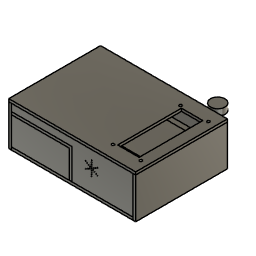
nfc_box (Autodesk Fusion 360 design; units mm, degrees)
Autodesk Fusion 360 part; units mm, degrees
note: some values were not read from the file. Chosen so that the rebuilt part matches the saved one: which bodies a step acts on. Set by a fixed rule: which sketch regions a step uses.
(part 1 of 2)
sketch "Sketch2" plane through (0, 0, 0) normal (0, 0, 1) x (1, 0, 0)
  line L0 (0, 0) -> (80, 0)
  line L1 (80, 0) -> (80, 36)
  line L2 (80, 36) -> (0, 36)
  line L3 (0, 36) -> (0, 0)
  line L4 (0, 0) -> (2.5, 0)
  line L5 (2.5, 0) -> (2.5, 2.5)
  line L6 (0, 0) -> (0, 5.6)
  line L7 (4.6, 5.6) -> (75.4, 5.6)
  line L8 (75.4, 5.6) -> (75.4, 29.4)
  line L9 (75.4, 29.4) -> (4.6, 29.4)
  line L10 (4.6, 29.4) -> (4.6, 5.6)
  circle A0 centre (2.5, 2.5) radius 1.5
  line L11 (0, 36) -> (2.5, 36)
  line L12 (80, 36) -> (77.5, 36)
  line L13 (80, 0) -> (80, 2.5)
  circle A1 centre (77.5, 33.5) radius 1.5
  circle A2 centre (77.5, 2.5) radius 1.5
  circle A3 centre (2.5, 33.5) radius 1.5
  line L14 (5.5434, 32.3445) -> (47.974, 32.3445)
  line L15 (47.974, 32.3445) -> (47.974, 35.1607)
  line L16 (47.974, 35.1607) -> (5.5434, 35.1607)
  line L17 (5.5434, 35.1607) -> (5.5434, 32.3445)
  dimension "d5" = 80
  dimension "d6" = 36
  dimension "d7" = 2.5
  dimension "d8" = 2.5
  dimension "d10" = 5.6
  dimension "d11" = 4.6
  dimension "d12" = 70.8
  dimension "d13" = 23.8
  dimension "d14" = 3
  dimension "d15" = 2.5
  dimension "d16" = 2.5
  dimension "d17" = 2.5
  dimension "d18" = 2.5
  dimension "d19" = 2.5
  dimension "d20" = 2.5
  dimension "d21" = 3
  dimension "d22" = 3
  dimension "d23" = 3
  constraint horizontal L0
  constraint vertical L1
  constraint horizontal L2
  constraint vertical L3
  constraint coincident L0.start L3.end
  constraint perpendicular L3 L4
  constraint perpendicular L4 L5
  constraint perpendicular L4 L6
  constraint horizontal L7
  constraint vertical L8
  constraint horizontal L9
  constraint vertical L10
  constraint coincident L5.end A0.centre
  constraint perpendicular L3 L11
  constraint perpendicular L1 L12
  constraint perpendicular L0 L13
  constraint horizontal L14
  constraint vertical L15
  constraint horizontal L16
  constraint vertical L17
  measures "d5" distance of L0.start L0.end
  measures "d6" distance of L0.start L2.end
  measures "d7" distance of L0.start L4.end
  measures "d8" distance of L4.end L5.end
  measures "d10" distance of L0.start L6.end
  measures "d11" distance of L6.end L7.start
  measures "d12" distance of L7.start L7.end
  measures "d13" distance of L7.start L9.end
  measures "d14" diameter of A0
  measures "d15" distance of L2.end L11.end
  measures "d16" distance of L11.end A3.centre
  measures "d17" distance of L1.end L12.end
  measures "d18" distance of L12.end A1.centre
  measures "d19" distance of L0.end L13.end
  measures "d20" distance of L13.end A2.centre
  measures "d21" diameter of A1
  measures "d22" diameter of A2
  measures "d23" diameter of A3
extrude "Extrude1" add sketch "Sketch2" against normal blind 20 contours L14 L15 L16 L17 makes body 1
extrude "Extrude2" add sketch "Sketch2" along normal blind 2 separate body makes body 2
extrude "Extrude3" add sketch "Sketch2" along normal blind 2 contours L14 L15 L16 L17 bodies 1 2
extrude "Extrude4" add sketch "Sketch2" along normal blind 10 contours L7 L8 L9 L10 bodies 1
sketch "Sketch3" plane through (0, 0, 0) normal (0, 0, 1) x (1, 0, 0)
  line L0 (0, 0) -> (0, -10)
  line L1 (0, -10) -> (119.888, -10)
  line L2 (119.888, -10) -> (119.888, -60.038)
  line L3 (119.888, -60.038) -> (0, -60.038)
  line L4 (0, -60.038) -> (0, -10)
  line L5 (0, -10) -> (5.08, -10)
  line L6 (0, -60.038) -> (5.08, -60.038)
  line L7 (119.888, -10) -> (114.808, -10)
  line L8 (119.888, -60.038) -> (114.808, -60.038)
  circle A0 centre (114.808, -54.958) radius 1.778
  circle A1 centre (114.808, -15.08) radius 1.75
  circle A2 centre (5.08, -15.08) radius 1.75
  circle A3 centre (5.08, -54.958) radius 1.75
  line L9 (0, -60.038) -> (69.85, -60.038)
  line L10 (69.85, -60.038) -> (69.85, -10)
  line L11 (115.1009, -20.75) -> (118.3077, -20.75)
  line L12 (118.3077, -20.75) -> (118.3077, -48.0699)
  line L13 (118.3077, -48.0699) -> (115.1009, -48.0699)
  line L14 (115.1009, -48.0699) -> (115.1009, -20.75)
  dimension "d32" = 10
  dimension "d33" = 119.888
  dimension "d34" = 50.038
  dimension "d35" = 5.08
  dimension "d36" = 5.08
  dimension "d37" = 5.08
  dimension "d38" = 5.08
  dimension "d39" = 5.08
  dimension "d40" = 5.08
  dimension "d41" = 5.08
  dimension "d42" = 5.08
  dimension "d44" = 3.5
  dimension "d45" = 3.5
  dimension "d46" = 3.5
  dimension "d47" = 69.85
  constraint coincident L0.start origin
  constraint vertical L0
  constraint horizontal L1
  constraint vertical L2
  constraint horizontal L3
  constraint vertical L4
  constraint perpendicular L0 L5
  constraint perpendicular L4 L6
  constraint perpendicular L2 L7
  constraint coincident L3 L8.end
  constraint coincident L1 L10.end
  constraint perpendicular L1 L10
  constraint horizontal L11
  constraint vertical L12
  constraint horizontal L13
  constraint vertical L14
  measures "d32" distance of L0.start L0.end
  measures "d33" distance of L0.end L1.end
  measures "d34" distance of L0.end L3.end
  measures "d35" distance of L0.end L5.end
  measures "d36" distance of L5.end A2.centre
  measures "d37" distance of L3.end L6.end
  measures "d38" distance of L6.end A3.centre
  measures "d39" distance of L1.end L7.end
  measures "d40" distance of L7.end A1.centre
  measures "d41" distance of L2.end L8.end
  measures "d42" distance of L8.end A0.centre
  measures "d44" diameter of A1
  measures "d45" diameter of A2
  measures "d46" diameter of A3
  measures "d47" distance of L3.end L9.end
extrude "Extrude5" add sketch "Sketch3" along normal blind 2 separate body makes body 3
extrude "Extrude6" add sketch "Sketch3" against normal blind 20 separate body contours L11 L12 L13 L14 makes body 4
extrude "Extrude7" add sketch "Sketch3" along normal blind 2 contours L11 L12 L13 L14 bodies 3 4
sketch "Sketch4" plane through (0, 0, 0) normal (0, 0, 1) x (1, 0, 0)
  circle A0 centre (109.1951, 29.6545) radius 8
  dimension "d54" = 16
  measures "d54" diameter of A0
extrude "Extrude8" add sketch "Sketch4" along normal blind 7 separate body makes body 5
sketch "Sketch5" plane through (0, 0, 0) normal (0, 0, 1) x (1, 0, 0)
  line L0 (-20, -18.2706) -> (-97, -18.2706)
  line L1 (-97, -18.2706) -> (-97, -68.2706)
  line L2 (-97, -68.2706) -> (-20, -68.2706)
  line L3 (-20, -68.2706) -> (-20, -18.2706)
  dimension "d58" = 77
  dimension "d59" = 50
  constraint horizontal L0
  constraint vertical L1
  constraint horizontal L2
  constraint vertical L3
  measures "d58" distance of L0.start L0.end
  measures "d59" distance of L0.start L2.end
extrude "Extrude9" add sketch "Sketch5" along normal blind 37 separate body makes body 6
extrude "Extrude10" cut 1 faces at (-71.3333, -34.9373, 37) along direction (0, 0, -1) blind 9 on bodies 6 bodies 6
sketch "Sketch6" plane through (0, 0, 0) normal (0, 0, 1) x (1, 0, 0)
  line L0 (0, 0) -> (-42.7427, 0)
  line L1 (-42.7427, 0) -> (-42.7427, 31.4009)
  line L2 (-42.7427, 31.4009) -> (0, 31.4009)
  line L3 (0, 31.4009) -> (0, 0)
  line L4 (-42.7427, 31.4009) -> (-133.7427, 31.4009)
  line L5 (-133.7427, 31.4009) -> (-133.7427, 93.4009)
  line L6 (-133.7427, 93.4009) -> (-42.7427, 93.4009)
  line L7 (-42.7427, 93.4009) -> (-42.7427, 31.4009)
  dimension "d64" = 91
  dimension "d65" = 62
  constraint horizontal L0
  constraint vertical L1
  constraint horizontal L2
  constraint vertical L3
  constraint coincident L0.start L3.end
  constraint horizontal L4
  constraint vertical L5
  constraint horizontal L6
  constraint vertical L7
  measures "d64" distance of L1.end L4.end
  measures "d65" distance of L1.end L6.end
extrude "Extrude11" add sketch "Sketch6" along normal blind 12 separate body contours L4 L5 L6 L7 makes body 7
move_body "Move1" bodies 1 to x (0, -1, 0) y (1, 0, 0) z (0, 0, 1) at (92.5, 5.5, 4)
move_body "Move2" bodies 1 to x (1, 0, 0) y (0, 1, 0) z (0, 0, 1) at (0, -1, 0)
move_body "Move3" bodies 1 to x (1, 0, 0) y (0, 1, 0) z (0, 0, 1) at (0, 0.5, 0)
move_body "Move4" bodies 6 to x (0, -1, 0) y (1, 0, 0) z (0, 0, 1) at (131.4465, -93.3947, -30)
move_body "Move5" bodies 7 to x (0, -1, 0) y (1, 0, 0) z (0, 0, 1) at (-32.9614, -123.5681, -20)
sketch "Sketch7" plane through (0, 0, -30) normal (0, 0, -1) x (1, 0, 0)
  line L0 (113.1759, 73.3947) -> (63.1759, 73.3947)
  line L1 (63.1759, 73.3947) -> (63.1759, -3.6053)
  line L2 (63.1759, -3.6053) -> (113.1759, -3.6053)
  line L3 (113.1759, -3.6053) -> (113.1759, 73.3947)
  line L4 (113.1759, -3.6053) -> (113.1759, -1.1053)
  line L5 (113.1759, -1.1053) -> (110.6759, -1.1053)
  line L6 (113.1759, -3.6053) -> (110.6759, -1.1053)
  line L7 (63.1759, 73.3947) -> (65.6762, 70.8944)
  line L8 (63.1759, 73.3947) -> (66.7119, 73.3947) construction
  line L9 (113.1759, 73.3947) -> (115.6762, 70.8944)
  line L10 (113.1759, 73.3947) -> (116.7119, 73.3947) construction
  line L11 (63.1759, -3.6053) -> (65.6762, -1.1049)
  line L12 (63.1759, -3.6053) -> (66.7119, -3.6053) construction
  circle A0 centre (65.6762, -1.1049) radius 1.5
  circle A1 centre (110.6759, -1.1053) radius 1.5
  circle A2 centre (65.6762, 70.8944) radius 1.5
  line L13 (113.1759, 73.3947) -> (110.6755, 70.8944)
  circle A3 centre (110.6755, 70.8944) radius 1.5
  dimension "d68" = 2.5
  dimension "d69" = 2.5
  dimension "d71" = 45
  dimension "d72" = 3.536
  dimension "d73" = 45
  dimension "d74" = 3.536
  dimension "d75" = 45
  dimension "d76" = 3.536
  dimension "d77" = 3
  dimension "d78" = 3
  dimension "d79" = 3
  dimension "d80" = 3.536
  dimension "d81" = 3
  constraint coincident L2.end L3.start
  constraint perpendicular L2 L4
  constraint perpendicular L4 L5
  constraint horizontal L8
  constraint coincident L0.end L1.start
  constraint horizontal L10
  constraint coincident L0.start L3.end
  constraint horizontal L12
  constraint coincident L1.end L2.start
  constraint coincident L11.end A0.centre
  constraint coincident L5.end L6.end
  constraint coincident L7.end A2.centre
  constraint perpendicular L9 L13
  constraint coincident L13.end A3.centre
  measures "d68" distance of L2.end L4.end
  measures "d69" distance of L4.end L5.end
  measures "d71" angle of L7 L8
  measures "d72" distance of L0.end L7.end
  measures "d73" angle of L9 L10
  measures "d74" distance of L0.start L9.end
  measures "d75" angle of L11 L12
  measures "d76" distance of L1.end L11.end
  measures "d77" diameter of A0
  measures "d78" diameter of A1
  measures "d79" diameter of A2
  measures "d80" distance of L0.start L13.end
  measures "d81" diameter of A3
extrude "Extrude12" cut sketch "Sketch7" against normal blind 44 contours L5 L6 A1 | L5 L6 A1 | A0 | A2 | A3 bodies 1 6
move_body "Move6" bodies 6 to x (1, 0, 0) y (0, 1, 0) z (0, 0, 1) at (0, 0, -4)
sketch "Sketch8" plane through (0, 0, -34) normal (0, 0, -1) x (1, 0, 0)
  circle A0 centre (65.6762, -1.1049) radius 1.5
  circle A1 centre (65.6762, 70.8944) radius 1.5
  circle A2 centre (110.6759, -1.1053) radius 1.5
  circle A3 centre (110.6755, 70.8944) radius 1.5
  line L0 (113.1759, 73.3947) -> (63.1759, 73.3947)
  line L1 (63.1759, 73.3947) -> (63.1759, -3.6053)
  line L2 (63.1759, -3.6053) -> (113.1759, -3.6053)
  line L3 (113.1759, -3.6053) -> (113.1759, 73.3947)
  line L4 (-1.5605, 80.8254) -> (60.4395, 80.8254)
  line L5 (-1.5605, -10.1746) -> (-1.5605, 80.8254)
  line L6 (60.4395, -10.1746) -> (-1.5605, -10.1746)
  line L7 (60.4395, 80.8254) -> (60.4395, -10.1746)
  circle A4 centre (5.08, 54.958) radius 1.75
  circle A5 centre (114.808, 15.08) radius 1.75
  circle A6 centre (5.08, 15.08) radius 1.75
  circle A7 centre (114.808, 54.958) radius 1.778
  line L8 (119.888, 10) -> (0, 10)
  line L9 (119.888, 60.038) -> (119.888, 10)
  line L10 (0, 60.038) -> (119.888, 60.038)
  line L11 (0, 10) -> (0, 60.038)
  circle A8 centre (65.6762, -1.1049) radius 1.5
  circle A9 centre (65.6762, 70.8944) radius 1.5
  circle A10 centre (110.6759, -1.1053) radius 1.5
  circle A11 centre (110.6755, 70.8944) radius 1.5
  line L12 (113.1759, 73.3947) -> (63.1759, 73.3947)
  line L13 (113.1759, -3.6053) -> (113.1759, 73.3947)
  line L14 (63.1759, -3.6053) -> (113.1759, -3.6053)
  line L15 (63.1759, 73.3947) -> (63.1759, -3.6053)
  arc A12 (109.352, -0.4) -> (111.9997, -0.4) centre (110.6759, -1.1053) ccw
  arc A13 (111.9997, -0.4) -> (109.352, -0.4) centre (110.6759, -1.1053) ccw
  arc A14 (112.0917, 70.4) -> (109.2594, 70.4) centre (110.6755, 70.8944) ccw
  arc A15 (109.2594, 70.4) -> (112.0917, 70.4) centre (110.6755, 70.8944) ccw
  circle A16 centre (95, -2.5) radius 1.5
  circle A17 centre (126, 72.5) radius 1.5
  circle A18 centre (95, 72.5) radius 1.5
  circle A19 centre (126, -2.5) radius 1.5
  line L16 (128.5, -5) -> (92.5, -5)
  line L17 (128.5, 75) -> (128.5, -5)
  line L18 (92.5, 75) -> (128.5, 75)
  line L19 (92.5, -5) -> (92.5, 75)
  line L20 (-1.5605, 80.8254) -> (-4.0608, 83.3257)
  line L21 (-1.5605, 80.8254) -> (1.9755, 80.8254) construction
  line L22 (128.5, -10.1746) -> (131.0003, -12.6749)
  line L23 (128.5, -10.1746) -> (132.036, -10.1746) construction
  line L24 (-4.0608, 83.3257) -> (131.0003, 83.3257)
  line L25 (131.0003, 83.3257) -> (131.0003, -12.6749)
  line L26 (131.0003, -12.6749) -> (-4.0608, -12.6749)
  line L27 (-4.0608, -12.6749) -> (-4.0608, 83.3257)
  line L28 (-7.0608, 83.3257) -> (-7.0608, 86.3257)
  line L29 (-7.0608, 86.3257) -> (-4.0608, 86.3257)
  line L30 (134.0003, -12.6749) -> (134.0003, -15.6749)
  line L31 (134.0003, -15.6749) -> (131.0003, -15.6749)
  line L32 (-7.0608, 86.3257) -> (134.0003, 86.3257)
  line L33 (134.0003, 86.3257) -> (134.0003, -15.6749)
  line L34 (134.0003, -15.6749) -> (-7.0608, -15.6749)
  line L35 (-7.0608, -15.6749) -> (-7.0608, 86.3257)
  dimension "d84" = 135
  dimension "d85" = 3.536
  dimension "d86" = 3.536
  dimension "d87" = 45
  dimension "d88" = 3
  dimension "d89" = 3
  dimension "d90" = 3
  dimension "d91" = 3
  constraint horizontal L21
  constraint coincident L4.start L5.end
  constraint horizontal L23
  constraint horizontal L24
  constraint vertical L25
  constraint horizontal L26
  constraint vertical L27
  constraint vertical L28
  constraint horizontal L29
  constraint vertical L30
  constraint horizontal L31
  constraint horizontal L32
  constraint vertical L33
  constraint horizontal L34
  constraint vertical L35
  measures "d84" angle of L20 L21
  measures "d85" distance of L4.start L20.end
  measures "d86" distance of L22.start L22.end
  measures "d87" angle of L22 L23
  measures "d88" distance of L20.end L28.start
  measures "d89" distance of L20.end L29.end
  measures "d90" distance of L22.end L30.start
  measures "d91" distance of L22.end L31.end
extrude "Extrude13" add sketch "Sketch8" against normal blind 42 separate body contours L28 L29 L30 L31 L32 L33 L34 L35 makes body 8
extrude "Extrude14" add sketch "Sketch8" along normal blind 3 contours L0 L3 L10 L12 L13 A18 L19 | L0 L2 L3 L8 L9 L10 L12 L13 L14 A16 A18 L16 L17 L18 L19 | L3 A5 A7 L8 L9 L10 L13 | L3 A5 A7 L8 L10 L13 L19 | L1 L8 L10 L15 L19 | L0 L1 L10 L12 L15 L19 | L1 L7 L8 L10 L15 | L1 L2 L8 L14 L15 L19 | L2 L3 L8 L13 L14 A16 L19 | L4 L5 L6 L7 L8 L10 L11 | L7 L8 L10 L11 | L24 L25 L26 L27 | L28 L29 L30 L31 L32 L33 L34 L35 bodies 6 8
extrude "Extrude15" add sketch "Sketch8" along normal blind 3 contours L0 L12 A18 | L0 L12 A18 | L2 L14 A16 | L2 L14 A16 | A17 | A19 bodies 6
extrude "Extrude16" add sketch "Sketch8" along normal blind 3 contours L3 A7 L13 | L3 A7 L13 | L3 A5 L13 | L3 A5 L13 | A4 | A6 bodies 6
sketch "Sketch9" plane through (0, -86.3257, 0) normal (0, -1, 0) x (1, 0, 0)
  line L0 (134.0003, -37) -> (134.0003, 8)
  line L1 (134.0003, 8) -> (-7.0608, 8)
  line L2 (-7.0608, 8) -> (-7.0608, -37)
  line L3 (-7.0608, -37) -> (134.0003, -37)
  circle A0 centre (84.9891, -10.0469) radius 8
  line L4 (84.9891, -10.0469) -> (84.9891, -2.0469)
  circle A1 centre (84.9891, -10.0469) radius 0.5
  circle A2 centre (84.9891, -8.1719) radius 0.5
  circle A3 centre (84.9891, -6.2969) radius 0.5
  circle A4 centre (84.9891, -4.4219) radius 0.5
  circle A5 centre (84.9891, -2.5469) radius 0.5
  circle A6 centre (84.9891, -10.0469) radius 0.5
  circle A7 centre (83.3653, -9.1094) radius 0.5
  circle A8 centre (81.7415, -8.1719) radius 0.5
  circle A9 centre (80.1177, -7.2344) radius 0.5
  circle A10 centre (78.4939, -6.2969) radius 0.5
  circle A11 centre (84.9891, -10.0469) radius 0.5
  circle A12 centre (83.3653, -10.9844) radius 0.5
  circle A13 centre (81.7415, -11.9219) radius 0.5
  circle A14 centre (80.1177, -12.8594) radius 0.5
  circle A15 centre (78.4939, -13.7969) radius 0.5
  circle A16 centre (84.9891, -10.0469) radius 0.5
  circle A17 centre (84.9891, -11.9219) radius 0.5
  circle A18 centre (84.9891, -13.7969) radius 0.5
  circle A19 centre (84.9891, -15.6719) radius 0.5
  circle A20 centre (84.9891, -17.5469) radius 0.5
  circle A21 centre (84.9891, -10.0469) radius 0.5
  circle A22 centre (86.6129, -10.9844) radius 0.5
  circle A23 centre (88.2367, -11.9219) radius 0.5
  circle A24 centre (89.8605, -12.8594) radius 0.5
  circle A25 centre (91.4843, -13.7969) radius 0.5
  circle A26 centre (84.9891, -10.0469) radius 0.5
  circle A27 centre (86.6129, -9.1094) radius 0.5
  circle A28 centre (88.2367, -8.1719) radius 0.5
  circle A29 centre (89.8605, -7.2344) radius 0.5
  circle A30 centre (91.4843, -6.2969) radius 0.5
  point P0 (84.9891, -10.0469)
  point P1 (84.9891, -10.0469)
  dimension "d100" = 16
  dimension "d101" = 1
  dimension "d104" = 0
  dimension "d105" = 7.5
  dimension "d107" = 360
  constraint coincident P1 P0
  constraint coincident A0 L4.end
  constraint vertical L4
  measures "d100" diameter of A0
  measures "d101" diameter of A1
extrude "Extrude17" cut sketch "Sketch9" against normal blind 5.5 contours A30 | L4 A5 | L4 A5 | A10 | A15 | A20 | A25 | L4 A2 | L4 A2 | L4 A3 | L4 A3 | L4 A4 | L4 A4 | A1 A6 A11 A16 A21 A26 | A7 | A8 | A9 | A12 | A13 | A14 | A17 | A18 | A19 | A22 | A23 | A24 | A27 | A28 | A29 bodies 6
sketch "Sketch10" plane through (0, 0, 8) normal (0, 0, 1) x (-1, 0, 0)
  line L0 (4.0608, -12.6749) -> (-131.0003, -12.6749)
  line L1 (-131.0003, -12.6749) -> (-131.0003, 83.3257)
  line L2 (-131.0003, 83.3257) -> (4.0608, 83.3257)
  line L3 (4.0608, 83.3257) -> (4.0608, -12.6749)
  line L4 (-134.0003, -15.6749) -> (7.0608, -15.6749)
  line L5 (7.0608, -15.6749) -> (7.0608, 86.3257)
  line L6 (7.0608, 86.3257) -> (-134.0003, 86.3257)
  line L7 (-134.0003, 86.3257) -> (-134.0003, -15.6749)
  line L8 (7.0608, -15.6749) -> (-134.0003, -15.6749)
  line L9 (-134.0003, -15.6749) -> (-134.0003, 86.3257)
  line L10 (-134.0003, 86.3257) -> (7.0608, 86.3257)
  line L11 (7.0608, 86.3257) -> (7.0608, -15.6749)
  arc A0 (-109.352, -0.4) -> (-111.9997, -0.4) centre (-110.6759, -1.1053) ccw
  line L12 (-109.352, -0.4) -> (-98.1, -0.4)
  line L13 (-98.1, -0.4) -> (-98.1, 70.4)
  line L14 (-98.1, 70.4) -> (-109.2594, 70.4)
  arc A1 (-112.0917, 70.4) -> (-109.2594, 70.4) centre (-110.6755, 70.8944) ccw
  line L15 (-112.0917, 70.4) -> (-121.9, 70.4)
  line L16 (-121.9, 70.4) -> (-121.9, -0.4)
  line L17 (-121.9, -0.4) -> (-111.9997, -0.4)
  circle A2 centre (-95, -2.5) radius 1.5
  circle A3 centre (-126, -2.5) radius 1.5
  circle A4 centre (-126, 72.5) radius 1.5
  circle A5 centre (-95, 72.5) radius 1.5
  constraint horizontal L8
  constraint vertical L9
  constraint horizontal L10
  constraint vertical L11
  constraint coincident L6.end L7.start
  constraint coincident L4.end L5.start
extrude "Extrude18" add sketch "Sketch10" along normal blind 3 separate body contours L0 L1 L2 L3 | L4 L5 L6 L7 L8 L9 L10 L11 makes body 9
sketch "Sketch11" plane through (0, 0, 11) normal (0, 0, 1) x (-1, 0, 0)
  circle A0 centre (-126, -2.5) radius 1.5
  circle A1 centre (-126, 72.5) radius 1.5
  circle A2 centre (-95, 72.5) radius 1.5
  line L0 (-121.9, 70.4) -> (-112.0917, 70.4)
  arc A3 (-112.0917, 70.4) -> (-109.2594, 70.4) centre (-110.6755, 70.8944) ccw
  line L1 (-109.2594, 70.4) -> (-98.1, 70.4)
  line L2 (-98.1, 70.4) -> (-98.1, -0.4)
  line L3 (-98.1, -0.4) -> (-109.352, -0.4)
  arc A4 (-109.352, -0.4) -> (-111.9997, -0.4) centre (-110.6759, -1.1053) ccw
  line L4 (-111.9997, -0.4) -> (-121.9, -0.4)
  line L5 (-121.9, -0.4) -> (-121.9, 70.4)
  circle A5 centre (-95, -2.5) radius 1.5
  line L6 (7.0608, 86.3257) -> (-134.0003, 86.3257)
  line L7 (-134.0003, 86.3257) -> (-134.0003, -15.6749)
  line L8 (-134.0003, -15.6749) -> (7.0608, -15.6749)
  line L9 (7.0608, -15.6749) -> (7.0608, 86.3257)
sketch "Sketch12" plane through (0, 0, 11) normal (0, 0, 1) x (-1, 0, 0)
  circle A0 centre (-126, -2.5) radius 1.5
  circle A1 centre (-126, 72.5) radius 1.5
  circle A2 centre (-95, 72.5) radius 1.5
  line L0 (-121.9, 70.4) -> (-112.0917, 70.4)
  arc A3 (-112.0917, 70.4) -> (-109.2594, 70.4) centre (-110.6755, 70.8944) ccw
  line L1 (-109.2594, 70.4) -> (-98.1, 70.4)
  line L2 (-98.1, 70.4) -> (-98.1, -0.4)
  line L3 (-98.1, -0.4) -> (-109.352, -0.4)
  arc A4 (-109.352, -0.4) -> (-111.9997, -0.4) centre (-110.6759, -1.1053) ccw
  line L4 (-111.9997, -0.4) -> (-121.9, -0.4)
  line L5 (-121.9, -0.4) -> (-121.9, 70.4)
  circle A5 centre (-95, -2.5) radius 1.5
  line L6 (7.0608, 86.3257) -> (-134.0003, 86.3257)
  line L7 (-134.0003, 86.3257) -> (-134.0003, -15.6749)
  line L8 (-134.0003, -15.6749) -> (7.0608, -15.6749)
  line L9 (7.0608, -15.6749) -> (7.0608, 86.3257)
  line L10 (-109.2594, 70.4) -> (-112.0917, 70.4)
  line L11 (-109.352, -0.4) -> (-111.9997, -0.4)
  line L12 (-111.9997, -0.4) -> (-111.9997, 1.5423)
  line L13 (-111.9997, 1.5423) -> (-109.7027, 1.5423)
  line L14 (-109.7027, 1.5423) -> (-109.352, -0.4)
  line L15 (-112.0917, 70.4) -> (-111.9997, 67.781)
  line L16 (-111.9997, 67.781) -> (-108.5038, 67.9037)
  line L17 (-108.5038, 67.9037) -> (-109.2594, 70.4)
  constraint coincident A3.end L1.start
  constraint coincident L0.end A3.start
  constraint coincident L3.end A4.start
  constraint coincident A4.end L4.start
  constraint perpendicular L4 L12
  constraint perpendicular L12 L13
  constraint perpendicular L15 L16
sketch "Sketch13" plane through (0, 0, 11) normal (0, 0, 1) x (-1, 0, 0)
extrude "Extrude19" cut sketch "Sketch12" against normal blind 3 contours A3 L10 | A4 L11 bodies 9
split "Split1" by plane through (131.0003, -83.3257, -34) normal (-1, 0, 0) bodies 6 makes body 10 at (16.794, -46.87, -37)
split "Split2" by plane through (131.0003, 12.6749, -34) normal (0, -1, 0) bodies 10 makes body 11 at (16.794, -47.87, -37)
split "Split3" by plane through (-4.0608, 12.6749, -34) normal (1, 0, 0) bodies 11 makes body 12 at (18.7564, -47.924, -37)
split "Split4" by plane through (0, 0, -34) normal (0, 0, 1) bodies 12 makes body 13 at (23.2908, -86.3257, -13.2656) makes body 14 at (95.4259, -23.3278, -6)
sketch "Sketch14" plane through (0, -86.3257, 0) normal (0, -1, 0) x (1, 0, 0)
  line L0 (131.0003, -34) -> (-4.0608, -34)
  line L1 (-4.0608, -34) -> (-4.0608, -37)
  line L2 (-4.0608, -37) -> (131.0003, -37)
  line L3 (131.0003, -37) -> (131.0003, -34)
  line L4 (113.1759, -6) -> (63.1759, -6)
  line L5 (63.1759, -6) -> (63.1759, -34)
  line L6 (63.1759, -34) -> (113.1759, -34)
  line L7 (113.1759, -34) -> (113.1759, -6)
  line L8 (0, 0) -> (119.888, 0)
  line L9 (119.888, 0) -> (119.888, 2)
  line L10 (119.888, 2) -> (0, 2)
  line L11 (0, 2) -> (0, 0)
  line L12 (63.1759, -34) -> (61.1759, -34)
  line L13 (63.1759, -34) -> (63.1759, 0)
  line L14 (63.1759, 0) -> (60.1759, 0)
  line L15 (60.1759, -3) -> (60.1759, -34)
  line L16 (60.1759, -34) -> (61.1759, -34)
  line L17 (-4.0608, -37) -> (-4.0608, 8)
  line L18 (-4.0608, 8) -> (-7.0608, 8)
  line L19 (-7.0608, 8) -> (-7.0608, -37)
  line L20 (-7.0608, -37) -> (-4.0608, -37)
  line L21 (-1.5605, -20) -> (60.4395, -20)
  line L22 (60.4395, -20) -> (60.4395, -8)
  line L23 (60.4395, -8) -> (-1.5605, -8)
  line L24 (-1.5605, -8) -> (-1.5605, -20)
  line L25 (0, 0) -> (-4.0608, 0)
  line L26 (-4.0608, 0) -> (-4.0608, -3)
  line L27 (-4.0608, -3) -> (60.1759, -3)
  dimension "d114" = 2
  dimension "d115" = 3
  dimension "d116" = 3
  constraint coincident L5.end L6.start
  constraint perpendicular L5 L12
  constraint coincident L8 L13.end
  constraint perpendicular L8 L13
  constraint perpendicular L13 L14
  constraint coincident L0 L15.end
  constraint perpendicular L0 L15
  constraint coincident L8.start L11.end
  constraint coincident L17 L25.end
  constraint perpendicular L17 L25
  constraint perpendicular L25 L26
  constraint perpendicular L15 L27
  measures "d114" distance of L5.end L12.end
  measures "d115" distance of L13.end L14.end
  measures "d116" distance of L25.end L26.end
extrude "Extrude20" add sketch "Sketch14" against normal up to surface (99.0007 mm away) separate body contours L0 L5 L8 L12 L13 L14 L15 L16 L17 L21 L22 L23 L25 L26 L27 | L15 L21 L22 L23 makes body 15
sketch "Sketch15" plane through (0, 0, 2) normal (0, 0, 1) x (-1, 0, 0)
  circle A0 centre (-114.808, 54.958) radius 1.778
  circle A1 centre (-5.08, 15.08) radius 1.75
  circle A2 centre (-114.808, 15.08) radius 1.75
  circle A3 centre (-5.08, 54.958) radius 1.75
  line L0 (0, 10) -> (0, 60.038)
  line L1 (0, 60.038) -> (-119.888, 60.038)
  line L2 (-119.888, 60.038) -> (-119.888, 10)
  line L3 (-119.888, 10) -> (0, 10)
  circle A4 centre (-5.08, 54.958) radius 1.75
  circle A5 centre (-5.08, 15.08) radius 1.75
extrude "Extrude21" cut sketch "Sketch15" against normal blind 15 contours A1 A5 | A3 A4 bodies 15
sketch "Sketch16" plane through (0, 3.6053, 0) normal (0, 1, 0) x (-1, 0, 0)
  line L0 (-63.1759, -6) -> (-113.1759, -6)
  line L1 (-113.1759, -6) -> (-113.1759, -34)
  line L2 (-113.1759, -34) -> (-63.1759, -34)
  line L3 (-63.1759, -34) -> (-63.1759, -6)
  line L4 (-88.1759, -34) -> (-88.1759, -20)
  line L5 (-113.1759, -20) -> (-88.1759, -20)
  line L6 (-82.1759, -25) -> (-94.1759, -25)
  line L7 (-94.1759, -25) -> (-94.1759, -15)
  line L8 (-94.1759, -15) -> (-82.1759, -15)
  line L9 (-82.1759, -15) -> (-82.1759, -25)
  line L10 (-82.1759, -25) -> (-94.1759, -15) construction
  line L11 (-94.1759, -25) -> (-82.1759, -15) construction
  point P0 (-88.1759, -20)
  dimension "d121" = 14
  dimension "d122" = 25
  dimension "d123" = 12
  dimension "d124" = 10
  constraint midpoint L2 L4.start
  constraint perpendicular L2 L4
  constraint midpoint L1 L5.start
  constraint perpendicular L1 L5
  constraint horizontal L6
  constraint perpendicular L6 L7
  constraint parallel L6 L8
  constraint parallel L7 L9
  constraint coincident L10 P0
  constraint coincident L11 P0
  constraint coincident P0 L4.end
  measures "d121" distance of L4.start P0
  measures "d122" distance of L5.start P0
  measures "d123" distance of L7.end L8.end
  measures "d124" distance of L6.end L7.end
ref_plane "WorkPlane1" through (0, 0, -55) normal (0, 0, 1) x (1, 0, 0)
sketch "bas" plane through (0, 0, -55) normal (0, 0, 1) x (1, 0, 0)
  circle A0 centre (65.6762, -70.8944) radius 1.5
  circle A1 centre (110.6755, -70.8944) radius 1.5
  circle A2 centre (110.6759, 1.1053) radius 1.5
  circle A3 centre (65.6762, 1.1049) radius 1.5
  line L0 (114.0003, -86.3257) -> (-7.0608, -86.3257)
  line L1 (-7.0608, -86.3257) -> (-7.0608, 15.6749)
  line L2 (12.9392, 15.6749) -> (114.0003, 15.6749)
  line L3 (134.0003, 15.6749) -> (134.0003, -86.3257)
  line L4 (-4.0608, -35.3254) -> (-4.0608, -45.3254)
  line L5 (-4.0608, -35.3254) -> (-4.0608, -25.3254)
  line L6 (-4.0608, -25.3254) -> (-7.0608, -25.3254)
  line L7 (-4.0608, -45.3254) -> (-7.0608, -45.3254)
  line L8 (-4.0608, -5.3254) -> (-4.0608, -15.3254)
  line L9 (-4.0608, -15.3254) -> (-7.0608, -15.3254)
  line L10 (-4.0608, -5.3254) -> (-4.0608, 4.6746)
  line L11 (-4.0608, 4.6746) -> (-7.0608, 4.6746)
  line L12 (-4.0608, -75.3254) -> (-7.0608, -75.3254)
  line L13 (-4.0608, -65.3254) -> (-4.0608, -75.3254)
  line L14 (-4.0608, -65.3254) -> (-4.0608, -55.3254)
  line L15 (-4.0608, -55.3254) -> (-7.0608, -55.3254)
  line L16 (131.0003, -35.3254) -> (131.0003, -45.3254)
  line L17 (131.0003, -35.3254) -> (131.0003, -25.3254)
  line L18 (131.0003, -25.3254) -> (134.0003, -25.3254)
  line L19 (131.0003, -45.3254) -> (134.0003, -45.3254)
  line L20 (131.0003, -15.3254) -> (134.0003, -15.3254)
  line L21 (131.0003, -5.3254) -> (131.0003, -15.3254)
  line L22 (131.0003, -5.3254) -> (131.0003, 4.6746)
  line L23 (131.0003, 4.6746) -> (134.0003, 4.6746)
  line L24 (131.0003, -75.3254) -> (134.0003, -75.3254)
  line L25 (131.0003, -65.3254) -> (131.0003, -75.3254)
  line L26 (131.0003, -65.3254) -> (131.0003, -55.3254)
  line L27 (131.0003, -55.3254) -> (134.0003, -55.3254)
  line L28 (60.1759, 12.6749) -> (63.1759, 12.6749)
  line L29 (63.1759, 12.6749) -> (63.1759, -86.3257)
  line L30 (63.1759, -86.3257) -> (60.1759, -86.3257)
  line L31 (60.1759, -86.3257) -> (60.1759, 12.6749)
  line L32 (60.1759, -45.3254) -> (63.1759, -45.3254)
  line L33 (60.1759, -25.3254) -> (63.1759, -25.3254)
  line L34 (60.1759, -55.3254) -> (63.1759, -55.3254)
  line L35 (60.1759, -75.3254) -> (63.1759, -75.3254)
  line L36 (60.1759, 4.6746) -> (63.1759, 4.6746)
  line L37 (60.1759, -15.3254) -> (63.1759, -15.3254)
  line L38 (63.1759, 4.6746) -> (63.1759, -15.3254)
  line L39 (60.1759, 4.6746) -> (60.1759, -15.3254)
  line L40 (63.1759, -25.3254) -> (63.1759, -45.3254)
  line L41 (60.1759, -25.3254) -> (60.1759, -45.3254)
  line L42 (63.1759, -55.3254) -> (63.1759, -75.3254)
  line L43 (60.1759, -75.3254) -> (60.1759, -55.3254)
  line L44 (134.0003, -86.3257) -> (114.0003, -86.3257)
  line L45 (60.1759, -86.3257) -> (80.1759, -86.3257)
  line L46 (114.0003, -86.3257) -> (114.0003, -83.3257)
  line L47 (134.0003, 15.6749) -> (114.0003, 15.6749)
  line L48 (114.0003, 15.6749) -> (114.0003, 12.6749)
  line L49 (114.0003, 12.6749) -> (84.0003, 12.6749)
  line L50 (84.0003, 12.6749) -> (84.0003, 15.6749)
  line L51 (-7.0608, 15.6749) -> (12.9392, 15.6749)
  line L52 (12.9392, 15.6749) -> (12.9392, 12.6749)
  line L53 (12.9392, 12.6749) -> (42.9392, 12.6749)
  line L54 (42.9392, 12.6749) -> (42.9392, 15.6749)
  circle A4 centre (110.6759, -63.8947) radius 1
  circle A5 centre (65.6762, -63.8947) radius 1
  circle A6 centre (110.6759, 1.1053) radius 1
  circle A7 centre (65.6762, 1.1049) radius 1
  line L55 (114.0003, -83.3257) -> (84.0003, -83.3257)
  line L56 (84.0003, -83.3257) -> (84.0003, -86.3257)
  circle A8 centre (76.6762, 6.1049) radius 1
  circle A9 centre (104.6762, 6.1049) radius 1
  point P0 (134.0003, -86.3257)
  point P1 (-7.0608, 15.6749)
  dimension "d127" = 10
  dimension "d128" = 10
  dimension "d131" = 0
  dimension "d132" = 30
  dimension "d135" = 0
  dimension "d136" = -30
  dimension "d138" = 10
  dimension "d139" = 10
  dimension "d142" = 0
  dimension "d143" = 30
  dimension "d146" = 0
  dimension "d147" = -30
  dimension "d148" = 20
  dimension "d149" = 20
  dimension "d151" = 3
  dimension "d152" = 20
  dimension "d153" = 3
  dimension "d154" = 30
  dimension "d155" = 20
  dimension "d156" = 3
  dimension "d157" = 30
  dimension "d233" = 2
  dimension "d234" = 2
  dimension "d235" = 2
  dimension "d236" = 2
  dimension "d237" = 30
  dimension "d240" = 2
  dimension "d241" = 28
  dimension "d242" = 2
  constraint horizontal L0
  constraint vertical L1
  constraint horizontal L2
  constraint vertical L3
  constraint coincident P1 L1.end
  constraint coincident P0 L3.end
  constraint coincident L1 L6.end
  constraint perpendicular L1 L6
  constraint coincident L1 L7.end
  constraint perpendicular L1 L7
  constraint coincident L3 L18.end
  constraint perpendicular L3 L18
  constraint coincident L3 L19.end
  constraint perpendicular L3 L19
  constraint coincident L29 L32.end
  constraint perpendicular L29 L32
  constraint coincident L29 L33.end
  constraint perpendicular L29 L33
  constraint coincident L31 L32.start
  constraint coincident L31 L33.start
  constraint coincident L29 L34.end
  constraint perpendicular L29 L34
  constraint coincident L29 L35.end
  constraint perpendicular L29 L35
  constraint coincident L29 L36.end
  constraint perpendicular L29 L36
  constraint coincident L29 L37.end
  constraint perpendicular L29 L37
  constraint coincident L31 L37.start
  constraint coincident L31 L36.start
  constraint coincident L31 L35.start
  constraint coincident L31 L34.start
  constraint perpendicular L3 L44
  constraint coincident L30.end L31.start
  constraint perpendicular L29 L45
  constraint perpendicular L44 L46
  constraint perpendicular L3 L47
  constraint perpendicular L2 L48
  constraint perpendicular L48 L49
  constraint coincident L2 L50.end
  constraint perpendicular L2 L50
  constraint perpendicular L1 L51
  constraint perpendicular L51 L52
  constraint perpendicular L52 L53
  constraint coincident L2 L54.end
  constraint perpendicular L2 L54
  constraint concentric A2 A6
  constraint concentric A3 A7
  constraint perpendicular L46 L55
  constraint coincident L0 L56.end
  constraint perpendicular L0 L56
  measures "d127" distance of L4.start L4.end
  measures "d128" distance of L4.start L5.end
  measures "d138" distance of L16.start L16.end
  measures "d139" distance of L16.start L17.end
  measures "d148" distance of P0 L0.start
  measures "d149" distance of L30.end L45.end
  measures "d151" distance of L0.start L46.end
  measures "d152" distance of L3.start L2.end
  measures "d153" distance of L2.end L48.end
  measures "d154" distance of L48.end L49.end
  measures "d155" distance of P1 L2.start
  measures "d156" distance of L2.start L52.end
  measures "d157" distance of L52.end L53.end
  measures "d233" diameter of A4
  measures "d234" diameter of A5
  measures "d235" diameter of A6
  measures "d236" diameter of A7
  measures "d237" distance of L46.end L55.end
  measures "d240" diameter of A8
  measures "d241" distance of A8.centre A9.centre
  measures "d242" diameter of A9
ref_plane "WorkPlane2" through (0, 0, 50) normal (0, 0, 1) x (1, 0, 0)
sketch "haut" plane through (0, 0, 50) normal (0, 0, 1) x (1, 0, 0)
  line L0 (-7.0608, -86.3257) -> (134.0003, -86.3257)
  line L1 (134.0003, -86.3257) -> (134.0003, 15.6749)
  line L2 (134.0003, 15.6749) -> (-7.0608, 15.6749)
  line L3 (-7.0608, 15.6749) -> (-7.0608, -86.3257)
  circle A0 centre (95, 2.5) radius 1.5
  circle A1 centre (95, -72.5) radius 1.5
  circle A2 centre (126, -72.5) radius 1.5
  circle A3 centre (126, 2.5) radius 1.5
  line L4 (98.1, 0.4) -> (121.9, 0.4)
  line L5 (121.9, 0.4) -> (121.9, -70.4)
  line L6 (121.9, -70.4) -> (98.1, -70.4)
  line L7 (98.1, -70.4) -> (98.1, 0.4)
  line L8 (114.0003, -83.3257) -> (80.1759, -83.3257)
  line L9 (80.1759, -86.3257) -> (80.1759, -83.3257)
  line L10 (114.0003, -86.3257) -> (114.0003, -83.3257)
  line L11 (114.0003, 15.6749) -> (114.0003, 12.6749)
  line L12 (114.0003, 12.6749) -> (84.0003, 12.6749)
  line L13 (84.0003, 12.6749) -> (84.0003, 15.6749)
  line L14 (42.9392, 12.6749) -> (42.9392, 15.6749)
  line L15 (12.9392, 12.6749) -> (42.9392, 12.6749)
  line L16 (12.9392, 15.6749) -> (12.9392, 12.6749)
  line L17 (-4.0608, -5.3254) -> (-4.0608, 4.6746)
  line L18 (-4.0608, 4.6746) -> (-7.0608, 4.6746)
  line L19 (-4.0608, -5.3254) -> (-4.0608, -15.3254)
  line L20 (-4.0608, -15.3254) -> (-7.0608, -15.3254)
  line L21 (-4.0608, -25.3254) -> (-7.0608, -25.3254)
  line L22 (-4.0608, -35.3254) -> (-4.0608, -25.3254)
  line L23 (-4.0608, -35.3254) -> (-4.0608, -45.3254)
  line L24 (-4.0608, -45.3254) -> (-7.0608, -45.3254)
  line L25 (-4.0608, -55.3254) -> (-7.0608, -55.3254)
  line L26 (-4.0608, -65.3254) -> (-4.0608, -55.3254)
  line L27 (-4.0608, -65.3254) -> (-4.0608, -75.3254)
  line L28 (-4.0608, -75.3254) -> (-7.0608, -75.3254)
  line L29 (131.0003, -75.3254) -> (134.0003, -75.3254)
  line L30 (131.0003, -65.3254) -> (131.0003, -75.3254)
  line L31 (131.0003, -65.3254) -> (131.0003, -55.3254)
  line L32 (131.0003, -55.3254) -> (134.0003, -55.3254)
  line L33 (131.0003, -15.3254) -> (134.0003, -15.3254)
  line L34 (131.0003, -5.3254) -> (131.0003, -15.3254)
  line L35 (131.0003, -5.3254) -> (131.0003, 4.6746)
  line L36 (131.0003, 4.6746) -> (134.0003, 4.6746)
  line L37 (131.0003, -25.3254) -> (134.0003, -25.3254)
  line L38 (131.0003, -35.3254) -> (131.0003, -25.3254)
  line L39 (131.0003, -35.3254) -> (131.0003, -45.3254)
  line L40 (131.0003, -45.3254) -> (134.0003, -45.3254)
  line L41 (63.1759, 4.6746) -> (63.1759, -15.3254)
  line L42 (60.1759, 4.6746) -> (60.1759, -15.3254)
  line L43 (60.1759, 4.6746) -> (63.1759, 4.6746)
  line L44 (60.1759, -15.3254) -> (63.1759, -15.3254)
  line L45 (60.1759, -25.3254) -> (63.1759, -25.3254)
  line L46 (63.1759, -25.3254) -> (63.1759, -45.3254)
  line L47 (60.1759, -25.3254) -> (60.1759, -45.3254)
  line L48 (60.1759, -45.3254) -> (63.1759, -45.3254)
  line L49 (63.1759, -55.3254) -> (63.1759, -75.3254)
  line L50 (60.1759, -75.3254) -> (63.1759, -75.3254)
  line L51 (60.1759, -75.3254) -> (60.1759, -55.3254)
  line L52 (60.1759, -55.3254) -> (63.1759, -55.3254)
  line L53 (12.9392, -86.3257) -> (12.9392, -83.3257)
  line L54 (12.9392, -83.3257) -> (42.9392, -83.3257)
  line L55 (42.9392, -83.3257) -> (42.9392, -86.3257)
  dimension "d159" = 20
  dimension "d160" = 3
  dimension "d161" = 30
  constraint vertical L53
  constraint perpendicular L53 L54
  constraint coincident L0 L55.end
  constraint perpendicular L0 L55
  measures "d159" distance of L0.start L53.start
  measures "d160" distance of L53.start L53.end
  measures "d161" distance of L53.end L54.end
ref_plane "WorkPlane3" through (0, -100, 0) normal (0, 1, 0) x (0, 0, 1)
sketch "son" plane through (0, -100, 0) normal (0, 1, 0) x (1, 0, 0)
  line L0 (-7.0608, -11) -> (134.0003, -11)
  line L1 (-7.0608, -8) -> (-7.0608, 37)
  line L2 (-7.0608, -8) -> (-7.0608, -11)
  line L3 (131.0003, 37) -> (-4.0608, 37)
  line L4 (-4.0608, 37) -> (-7.0608, 37)
  line L5 (134.0003, 37) -> (131.0003, 37)
  line L6 (134.0003, -8) -> (134.0003, 37)
  line L7 (134.0003, -8) -> (134.0003, -11)
  line L8 (114.0003, -8) -> (114.0003, -11)
  line L9 (84.0003, -11) -> (84.0003, -8)
  line L10 (-7.0608, -8) -> (12.9392, -8)
  line L11 (12.9392, -8) -> (12.9392, -11)
  line L12 (42.9392, -11) -> (42.9392, -8)
  line L13 (42.9392, -8) -> (44.6718, -8)
  line L14 (44.6718, -8) -> (84.0003, -8)
  line L15 (114.0003, -8) -> (115.1828, -8)
  line L16 (115.1828, -8) -> (134.0003, -8)
  line L17 (114.0003, 34) -> (114.0003, 37)
  line L18 (84.0003, 34) -> (84.0003, 37)
  line L19 (42.9392, 34) -> (42.9392, 37)
  line L20 (12.9392, 34) -> (12.9392, 37)
  line L21 (114.0003, 34) -> (134.0003, 34)
  line L22 (-7.0608, 34) -> (12.9392, 34)
  line L23 (42.9392, 34) -> (84.0003, 34)
  line L24 (-4.0608, 34) -> (131.0003, 34)
  line L25 (131.0003, 34) -> (131.0003, -8)
  line L26 (131.0003, -8) -> (-4.0608, -8)
  line L27 (-4.0608, -8) -> (-4.0608, 34)
  circle A0 centre (91.4843, 13.7969) radius 0.5
  circle A1 centre (91.4843, 6.2969) radius 0.5
  circle A2 centre (84.9891, 4.4219) radius 0.5
  circle A3 centre (84.9891, 10.0469) radius 0.5
  circle A4 centre (84.9891, 17.5469) radius 0.5
  circle A5 centre (83.3653, 9.1094) radius 0.5
  circle A6 centre (84.9891, 2.5469) radius 0.5
  circle A7 centre (81.7415, 8.1719) radius 0.5
  circle A8 centre (80.1177, 12.8594) radius 0.5
  circle A9 centre (84.9891, 11.9219) radius 0.5
  circle A10 centre (84.9891, 6.2969) radius 0.5
  circle A11 centre (89.8605, 7.2344) radius 0.5
  circle A12 centre (89.8605, 12.8594) radius 0.5
  circle A13 centre (86.6129, 10.9844) radius 0.5
  circle A14 centre (86.6129, 9.1094) radius 0.5
  circle A15 centre (78.4939, 13.7969) radius 0.5
  circle A16 centre (84.9891, 15.6719) radius 0.5
  circle A17 centre (83.3653, 10.9844) radius 0.5
  circle A18 centre (78.4939, 6.2969) radius 0.5
  circle A19 centre (80.1177, 7.2344) radius 0.5
  circle A20 centre (81.7415, 11.9219) radius 0.5
  circle A21 centre (84.9891, 13.7969) radius 0.5
  circle A22 centre (84.9891, 8.1719) radius 0.5
  circle A23 centre (88.2367, 8.1719) radius 0.5
  circle A24 centre (88.2367, 11.9219) radius 0.5
  line L28 (63.1759, 0) -> (-4.0608, 0)
  line L29 (-4.0608, 0) -> (-4.0608, 3)
  line L30 (-4.0608, 3) -> (60.1759, 3)
  line L31 (60.1759, 3) -> (60.1759, 34)
  line L32 (60.1759, 34) -> (63.1759, 34)
  line L33 (63.1759, 34) -> (63.1759, 0)
  line L34 (60.1759, 34) -> (60.1759, 37)
  line L35 (60.1759, 34) -> (60.1759, 31)
  line L36 (60.1759, 31) -> (-4.0608, 31)
  dimension "d163" = 20
  dimension "d164" = 30
  dimension "d165" = 20
  dimension "d166" = 30
  dimension "d167" = 3
  dimension "d168" = 3
  dimension "d170" = 3
  constraint coincident L6.start L7.start
  constraint coincident L0 L8.end
  constraint perpendicular L0 L8
  constraint coincident L1.start L2.start
  constraint perpendicular L2 L10
  constraint coincident L0 L11.end
  constraint perpendicular L0 L11
  constraint perpendicular L12 L13
  constraint perpendicular L9 L14
  constraint perpendicular L7 L16
  constraint coincident L3 L17.end
  constraint perpendicular L3 L17
  constraint perpendicular L14 L18
  constraint coincident L3 L19.end
  constraint perpendicular L3 L19
  constraint coincident L3 L20.end
  constraint perpendicular L3 L20
  constraint coincident L6 L21.end
  constraint perpendicular L6 L22
  constraint coincident L17.start L22
  constraint collinear L21 L22
  constraint collinear L22 L23
  constraint coincident L31.end L32.start
  constraint coincident L3 L34.end
  constraint perpendicular L3 L34
  constraint perpendicular L32 L35
  constraint coincident L27 L36.end
  constraint perpendicular L27 L36
  measures "d163" distance of L6.start L8.start
  measures "d164" distance of L8.end L9.start
  measures "d165" distance of L1.start L10.end
  measures "d166" distance of L11.end L12.start
  measures "d167" distance of L12.start L12.end
  measures "d168" distance of L1.end L22.start
  measures "d170" distance of L31.end L35.end
ref_plane "WorkPlane4" through (0, 60, 0) normal (0, 1, 0) x (0, 0, 1)
sketch "branchement" plane through (0, 60, 0) normal (0, 1, 0) x (1, 0, 0)
  line L0 (44.6718, -8) -> (84.0003, -8)
  line L1 (42.9392, -8) -> (44.6718, -8)
  line L2 (42.9392, -11) -> (42.9392, -8)
  line L3 (-7.0608, -11) -> (134.0003, -11)
  line L4 (12.9392, -8) -> (12.9392, -11)
  line L5 (-7.0608, -8) -> (12.9392, -8)
  line L6 (-7.0608, -8) -> (-7.0608, 37)
  line L7 (-7.0608, 34) -> (12.9392, 34)
  line L8 (12.9392, 34) -> (12.9392, 37)
  line L9 (131.0003, 37) -> (-4.0608, 37)
  line L10 (42.9392, 34) -> (42.9392, 37)
  line L11 (42.9392, 34) -> (84.0003, 34)
  line L12 (84.0003, 34) -> (84.0003, 37)
  line L13 (114.0003, 34) -> (114.0003, 37)
  line L14 (114.0003, 34) -> (134.0003, 34)
  line L15 (134.0003, -8) -> (134.0003, 37)
  line L16 (115.1828, -8) -> (134.0003, -8)
  line L17 (114.0003, -8) -> (114.0003, -11)
  line L18 (114.0003, -8) -> (115.1828, -8)
  line L19 (84.0003, -11) -> (84.0003, -8)
  line L20 (94.1759, 15) -> (82.1759, 15)
  line L21 (82.1759, 15) -> (82.1759, 25)
  line L22 (82.1759, 25) -> (94.1759, 25)
  line L23 (94.1759, 25) -> (94.1759, 15)
  line L24 (94.9869, 20) -> (82.9869, 20)
  line L25 (82.9869, 20) -> (82.9869, 10)
  line L26 (82.9869, 10) -> (94.9869, 10)
  line L27 (94.9869, 10) -> (94.9869, 20)
  dimension "d226" = 12
  dimension "d227" = 10
  constraint horizontal L24
  constraint vertical L25
  constraint horizontal L26
  constraint vertical L27
  measures "d226" distance of L24.start L24.end
  measures "d227" distance of L24.start L26.end
ref_plane "WorkPlane5" through (0, -140, 0) normal (0, 1, 0) x (1, 0, 0)
sketch "Sketch21" plane through (0, -140, 0) normal (0, 1, 0) x (1, 0, 0)
  line L0 (-7.0608, -11) -> (134.0003, -11)
  line L1 (131.0003, 37) -> (-4.0608, 37)
  line L2 (134.0003, 37) -> (131.0003, 37)
  line L3 (134.0003, -8) -> (134.0003, 37)
  line L4 (134.0003, -8) -> (134.0003, -11)
  line L5 (-7.0608, -8) -> (-7.0608, -11)
  line L6 (-7.0608, -8) -> (-7.0608, 37)
  line L7 (-4.0608, 37) -> (-7.0608, 37)
  line L8 (63.1759, 0) -> (-4.0608, 0)
  line L9 (63.1759, 34) -> (63.1759, 0)
  line L10 (60.1759, 34) -> (60.1759, 37)
  line L11 (60.1759, 34) -> (60.1759, 31)
  line L12 (60.1759, 3) -> (60.1759, 34)
  line L13 (-4.0608, 3) -> (60.1759, 3)
  line L14 (-7.0608, -8) -> (12.9392, -8)
  line L15 (12.9392, -8) -> (12.9392, -11)
  line L16 (44.6718, -8) -> (84.0003, -8)
  line L17 (42.9392, -8) -> (44.6718, -8)
  line L18 (42.9392, -11) -> (42.9392, -8)
  line L19 (84.0003, -11) -> (84.0003, -8)
  line L20 (114.0003, -8) -> (114.0003, -11)
  line L21 (115.1828, -8) -> (134.0003, -8)
  line L22 (114.0003, -8) -> (115.1828, -8)
  line L23 (114.0003, 34) -> (134.0003, 34)
  line L24 (114.0003, 34) -> (114.0003, 37)
  line L25 (84.0003, 34) -> (84.0003, 37)
  circle A0 centre (84.9891, 17.5469) radius 0.5
  circle A1 centre (84.9891, 15.6719) radius 0.5
  circle A2 centre (84.9891, 13.7969) radius 0.5
  circle A3 centre (84.9891, 11.9219) radius 0.5
  circle A4 centre (84.9891, 10.0469) radius 0.5
  circle A5 centre (84.9891, 8.1719) radius 0.5
  circle A6 centre (84.9891, 6.2969) radius 0.5
  circle A7 centre (84.9891, 4.4219) radius 0.5
  circle A8 centre (84.9891, 2.5469) radius 0.5
  circle A9 centre (91.4843, 6.2969) radius 0.5
  circle A10 centre (89.8605, 7.2344) radius 0.5
  circle A11 centre (88.2367, 8.1719) radius 0.5
  circle A12 centre (86.6129, 9.1094) radius 0.5
  circle A13 centre (86.6129, 10.9844) radius 0.5
  circle A14 centre (88.2367, 11.9219) radius 0.5
  circle A15 centre (89.8605, 12.8594) radius 0.5
  circle A16 centre (91.4843, 13.7969) radius 0.5
  circle A17 centre (83.3653, 9.1094) radius 0.5
  circle A18 centre (81.7415, 8.1719) radius 0.5
  circle A19 centre (80.1177, 7.2344) radius 0.5
  circle A20 centre (78.4939, 6.2969) radius 0.5
  circle A21 centre (83.3653, 10.9844) radius 0.5
  circle A22 centre (81.7415, 11.9219) radius 0.5
  circle A23 centre (80.1177, 12.8594) radius 0.5
  circle A24 centre (78.4939, 13.7969) radius 0.5
  line L26 (-4.0608, 3) -> (-4.0608, 31)
  line L27 (60.1759, 31) -> (-4.0608, 31)
  line L28 (84.0003, 34) -> (63.1759, 34)
  line L29 (63.1759, 34) -> (60.1759, 34)
  line L30 (60.1759, 34) -> (-4.0608, 34)
  line L31 (-4.0608, 34) -> (-4.0608, 31)
  constraint coincident L13.start L26.start
  constraint perpendicular L13 L26
  constraint coincident L11.end L27.start
  constraint perpendicular L26 L27
  constraint coincident L25.start L28.start
  constraint coincident L9.start L28.end
  constraint coincident L10.start L11.start
  constraint perpendicular L6 L30
  constraint perpendicular L27 L31
ref_plane "WorkPlane6" through (160, 0, 0) normal (1, 0, 0) x (0, 1, 0)